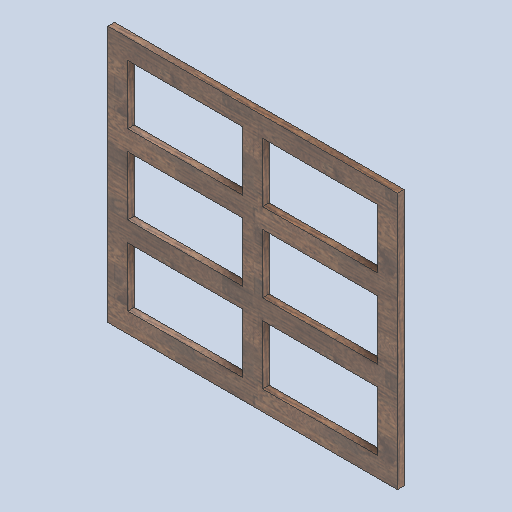
# Autodesk Inventor part: Front Panel
Saved by Autodesk Inventor 2022 (Build 260153000, 153)
## iProperties
Created: 2021-10-04
Part Number: Front Panel
Material: Generic
Document SubType Name: Modeling
Designer: Admin
Density: 1 g/cm^3
Appearance: White Ash - Java
Author: Admin
Autodesk Inventor part; units mm, degrees
ref_plane "YZ Plane" through (0, 0, 0) normal (1, 0, 0) x (0, 1, 0)
ref_plane "XZ Plane" through (0, 0, 0) normal (0, 1, 0) x (-1, 0, 0)
ref_plane "XY Plane" through (0, 0, 0) normal (0, 0, 1) x (1, 0, 0)
derived "Dresser SKELETON.ipt"
sketch "Front Panel Sketch" plane through (0, 0, 342.9) normal (0, 0, 1) x (1, 0, 0)
  line L0 (558.8, 152.4) -> (-558.8, 152.4)
  line L1 (-558.8, 152.4) -> (-558.8, 1143)
  line L2 (-558.8, 1143) -> (558.8, 1143)
  line L3 (558.8, 1143) -> (558.8, 152.4)
  line L4 (635, 1219.2) -> (-635, 1219.2) construction
  point P0 (0, 0)
  point P1 (0, 152.4)
  point P2 (-558.8, 0)
  point P3 (-558.8, 0)
  point P4 (-558.8, 0)
  point P5 (558.8, 0)
  point P6 (558.8, 0)
  point P7 (558.8, 0)
  dimension "panelWidth" = 1117.6
  measures "panelWidth" distance of L0.start L0.end
sketch "Drawer Cut Sketch" plane through (0, 0, 342.9) normal (0, 0, 1) x (1, 0, 0)
  line L0 (-558.8, 152.4) -> (-558.8, 1143) construction
  line L1 (558.8, 152.4) -> (-558.8, 152.4) construction
  line L2 (-482.6, 228.6) -> (-38.1, 228.6)
  line L3 (-38.1, 228.6) -> (-38.1, 457.2)
  line L4 (-38.1, 457.2) -> (-482.6, 457.2)
  line L5 (-482.6, 457.2) -> (-482.6, 228.6)
  point P0 (0, 0)
extrude "Extrusion1" add sketch "Front Panel Sketch" along normal blind 25.4
extrude "Extrusion2" cut sketch "Drawer Cut Sketch" along normal blind 25.4
pattern_linear "Rectangular Pattern1" count 2 spacing 520.7 along (1, 0, 0) count 3 spacing 304.8 along (0, 1, 0) of "Extrusion2"
equation "\"d1\" = panelThickness"
equation "\"d3\" = panelThickness"
equation "\"rowSpacing\" = drawerHeight + drawerHorizontalOffset"
equation "\"columnSpacing\" = drawerWidth + drawerVerticalOffset"
equation "\"panelThickness\" = 25.4"
equation "\"drawerHeight\" = 228.6"
equation "\"drawerHorizontalOffset\" = 76.2"
equation "\"drawerWidth\" = 444.5"
equation "\"drawerVerticalOffset\" = 76.2"
body "Solid1"
